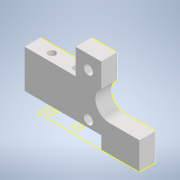
# Autodesk Inventor part: MotorHolder 2
Saved by Autodesk Inventor 2020.1 (Build 241239000, 239)
## iProperties
Created: 2019-10-30
Part Number: MotorHolder 2
Material: Generic
Document SubType Name: Modeling
Designer: j8qin
Density: 1 g/cm^3
Appearance: Default
Author: j8qin
Autodesk Inventor part; units mm, degrees
ref_plane "YZ Plane" through (0, 0, 0) normal (1, 0, 0) x (0, 1, 0)
ref_plane "XZ Plane" through (0, 0, 0) normal (0, 1, 0) x (-1, 0, 0)
ref_plane "XY Plane" through (0, 0, 0) normal (0, 0, 1) x (1, 0, 0)
sketch "Sketch1" plane through (0, 0, 0) normal (0, 0, 1) x (1, 0, 0)
  line L0 (0, 0) -> (25.4, 0)
  line L1 (25.4, 25.4) -> (15.24, 25.4)
  line L2 (15.24, 25.4) -> (15.24, 15.24)
  line L3 (15.24, 15.24) -> (0, 15.24)
  line L4 (0, 15.24) -> (0, 0)
  line L5 (20.32, 25.4) -> (20.32, 0) construction
  circle A0 centre (20.32, 2.75) radius 1.7907
  circle A1 centre (20.32, 19.95) radius 1.7907
  arc A2 (25.4, 15.8417) -> (28.612, 5.828) centre (28.612, 11.35) ccw
  line L6 (40.64, -5.08) -> (25.4, -5.08)
  line L7 (25.4, -5.08) -> (25.4, 0)
  line L8 (25.4, 0) -> (25.4, 6.8583) construction
  line L9 (25.4, 15.8417) -> (25.4, 25.4)
  line L10 (28.612, 5.828) -> (40.64, 5.828)
  line L11 (40.64, 5.828) -> (40.64, -5.08)
  dimension "d0" = 25.4
  dimension "d1" = 25.4
  dimension "d2" = 10.16
  dimension "d3" = 10.16
  dimension "d4" = 3.5814
  dimension "d6" = 2.75
  dimension "d7" = 3.5814
  dimension "d17" = 17.2
  dimension "d18" = 11.044
  dimension "d20" = 11.35
  dimension "d21" = 8.292
  dimension "d24" = 15.24
  dimension "d25" = 5.08
  dimension "d26" = 15.24
  constraints: 24 end point, 9 perpendicular, 3 centre point, 3 point on circle, 3 point on line, 1 horizontal, 1 midpoint, 1 vertical
  measures "d0" distance of L0.start L0.end
  measures "d1" distance of L0.end L1.start
  measures "d2" distance of L1.start L1.end
  measures "d3" distance of L1.end L2.end
  measures "d4" diameter of A0
  measures "d6" distance from line of L0 A0.centre
  measures "d7" diameter of A1
  measures "d17" distance of A0.centre A1.centre
  measures "d18" diameter of A2
  measures "d20" distance from line of L0 A2.centre
  measures "d21" horizontal distance of A1.centre A2.centre
  measures "d24" distance of L6.start L6.end
  measures "d25" distance of L6.end L0.end
  measures "d26" distance between parallel lines of L4 L2
extrude "Extrusion1" add sketch "Sketch1" along normal mid plane 6.35
sketch "Sketch2" plane through (0, 15.24, 3.175) normal (0, 1, 0) x (1, 0, 0)
  line L0 (0, 3.175) -> (15.24, 3.175) construction
  line L1 (15.24, 6.35) -> (15.24, 0) projected
  circle A0 centre (2.54, 3.175) radius 1.4605
  circle A1 centre (12.7, 3.175) radius 1.4605
  line L2 (0, 6.35) -> (0, 0) projected
  dimension "d11" = 2.921
  dimension "d12" = 2.921
  dimension "d13" = 2.54
  dimension "d14" = 12.7
  constraints: 2 centre point, 2 end point, 2 point on line, 1 midpoint
  measures "d11" diameter of A0
  measures "d12" diameter of A1
  measures "d13" distance from line of L2 A0.centre
  measures "d14" distance from line of L2 A1.centre
extrude "Extrusion2" cut sketch "Sketch2" against normal up to next
sketch "Sketch4" plane through (25.4, -5.08, 3.175) normal (0, -1, 0) x (1, 0, 0)
  circle A0 centre (-22.86, -3.175) radius 1.4605 projected
  circle A1 centre (-12.7, -3.175) radius 1.4605 projected
  line L0 (0, -6.35) -> (0, 0) projected
  line L1 (-25.4, 0) -> (0, 0) projected
  line L2 (-25.4, 0) -> (-25.4, -6.35) projected
  line L3 (0, -6.35) -> (-25.4, -6.35) projected
  line L4 (15.24, -6.35) -> (15.24, 0) projected
  line L5 (0, 0) -> (15.24, 0) projected
  line L6 (0, -6.35) -> (0, 0) projected
  line L7 (15.24, -6.35) -> (0, -6.35) projected
  point P0 (-25.4, -3.175)
sketch "Sketch5" plane through (0, 0, 3.175) normal (-1, 0, 0) x (0, 0, 1)
  line L0 (0, 0) -> (-6.35, 0) projected
  line L1 (0, 15.24) -> (0, 0) projected
  line L2 (-6.35, 15.24) -> (0, 15.24) projected
  line L3 (-6.35, 0) -> (-6.35, 15.24) projected
  point P0 (-3.175, 0)
extrude "Extrusion3" add sketch "Sketch5" along normal blind 5.08
sketch "Sketch6" plane through (0, 0, -3.175) normal (0, 0, -1) x (-1, 0, 0)
  circle A0 centre (-20.32, 19.95) radius 1.7907 projected
  circle A1 centre (-20.32, 2.75) radius 1.7907 projected
  line L0 (-25.4, 0) -> (5.08, 0) projected
  line L1 (5.08, 15.24) -> (5.08, 0) projected
  line L2 (-15.24, 15.24) -> (5.08, 15.24) projected
  line L3 (-15.24, 15.24) -> (-15.24, 25.4) projected
  line L4 (-15.24, 25.4) -> (-25.4, 25.4) projected
  line L5 (-25.4, 25.4) -> (-25.4, 15.8417) projected
  arc A2 (-28.612, 5.828) -> (-25.4, 15.8417) centre (-28.612, 11.35) ccw projected
  line L6 (-28.612, 5.828) -> (-40.64, 5.828) projected
  line L7 (-40.64, 5.828) -> (-40.64, -5.08) projected
  line L8 (-40.64, -5.08) -> (-25.4, -5.08) projected
  line L9 (-25.4, -5.08) -> (-25.4, 0) projected
  line L10 (-11.2395, 15.24) -> (-11.2395, 0) projected
  line L11 (-11.2395, 15.24) -> (-11.2395, 0)
  line L12 (-14.1605, 15.24) -> (-11.2395, 15.24) projected
  line L13 (-14.1605, 15.24) -> (-14.1605, 0)
  line L14 (-25.4, 0) -> (5.08, 0) projected
  line L15 (-4.0005, 15.24) -> (-1.0795, 15.24) projected
  line L16 (-1.0795, 15.24) -> (-1.0795, 0)
  line L17 (-4.0005, 15.24) -> (-4.0005, 0)
  line L18 (-4.0005, 15.24) -> (-4.0005, 0) projected
  constraints: 8 end point, 8 point on line, 1 perpendicular, 1 vertical
body "Solid1"
